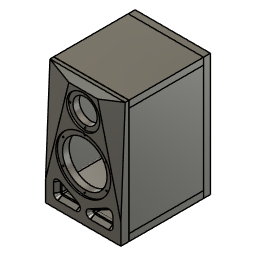
Spookers V2 v19 (Autodesk Fusion 360 design; units mm, degrees)
Autodesk Fusion 360 part; units mm, degrees
ref_plane "Arbeitsebene4" through (0, 0, 10) normal (0, 0, 1) x (1, 0, 0) in component "Front"
sketch "Skizze1" plane through (0, 0, 10) normal (0, 0, 1) x (1, 0, 0) in component "Front"
  line L0 (0, 0) -> (208, 0)
  line L1 (208, 0) -> (208, 338)
  line L2 (208, 338) -> (0, 338)
  line L3 (0, 338) -> (0, 0)
  line L4 (19, 319) -> (189, 319) construction
  line L5 (189, 319) -> (189, 19) construction
  line L6 (189, 19) -> (19, 19) construction
  line L7 (19, 19) -> (19, 319) construction
  line L8 (104, 0) -> (104, 338) construction
  circle A0 centre (104, 269.25) radius 33.5
  circle A1 centre (104, 269.25) radius 45.75
  circle A2 centre (104, 142.75) radius 75.75
  circle A3 centre (104, 142.75) radius 61.5
  line L9 (86.352941, 38.411765) -> (36.352941, 65.078431)
  line L10 (29, 60.666667) -> (29, 34)
  line L11 (34, 29) -> (84, 29)
  arc A4 (84, 29) -> (86.352941, 38.411765) centre (84, 34) ccw
  arc A5 (36.352941, 65.078431) -> (29, 60.666667) centre (34, 60.666667) ccw
  arc A6 (29, 34) -> (34, 29) centre (34, 34) ccw
  line L12 (121.647059, 38.411765) -> (171.647059, 65.078431)
  arc A7 (179, 60.666667) -> (171.647059, 65.078431) centre (174, 60.666667) ccw
  line L13 (179, 60.666667) -> (179, 34)
  arc A8 (174, 29) -> (179, 34) centre (174, 34) ccw
  line L14 (174, 29) -> (124, 29)
  arc A9 (121.647059, 38.411765) -> (124, 29) centre (124, 34) ccw
  circle A10 centre (104, 142.75) radius 69 construction
  circle A11 centre (104, 269.25) radius 41 construction
  circle A12 centre (104, 211.75) radius 2
  circle A13 centre (44.244247, 177.25) radius 2
  circle A14 centre (44.244247, 108.25) radius 2
  circle A15 centre (104, 73.75) radius 2
  circle A16 centre (163.755753, 108.25) radius 2
  circle A17 centre (163.755753, 177.25) radius 2
  circle A18 centre (104, 310.25) radius 2
  circle A19 centre (63, 269.25) radius 2
  circle A20 centre (104, 228.25) radius 2
  circle A21 centre (145, 269.25) radius 2
  point P0 (29, 69)
  point P1 (29, 29)
  dimension "d20" = 338
  dimension "d21" = 208
  dimension "d22" = 19
  dimension "d23" = 19
  dimension "d24" = 19
  dimension "d25" = 19
  dimension "d26" = 67
  dimension "d27" = 91.5
  dimension "d28" = 151.5
  dimension "d29" = 123
  dimension "d30" = 126.5
  dimension "d31" = 49.75
  dimension "d32" = 5
  dimension "d33" = 40
  dimension "d34" = 55
  dimension "d35" = 10
  dimension "d36" = 10
  dimension "d37" = 5
  dimension "d75" = 138
  dimension "d76" = 82
  dimension "d82" = 4
  dimension "d84" = 360
  dimension "d85" = 4
  dimension "d87" = 360
  constraint horizontal L0
  constraint vertical L1
  constraint horizontal L2
  constraint vertical L3
  constraint coincident L0.start L3.end
  constraint horizontal L4
  constraint vertical L5
  constraint horizontal L6
  constraint vertical L7
  constraint midpoint L0 L8.start
  constraint midpoint L2 L8.end
  constraint coincident L8 A0.centre
  constraint concentric A0 A1
  constraint coincident L8 A2.centre
  constraint concentric A2 A3
  constraint vertical L10
  constraint perpendicular L10 L11
  constraint tangent L11 A4
  constraint tangent L9 A4
  constraint coincident P0 L10
  constraint coincident P0 L9
  constraint tangent L10 A5
  constraint tangent L9 A5
  constraint coincident P1 L10
  constraint coincident P1 L11
  constraint tangent L10 A6
  constraint tangent L11 A6
  constraint equal A5 A6
  constraint symmetric L8 L11.end L14.end
  constraint symmetric L8 A4 A9
  constraint symmetric L8 A5 A7
  constraint symmetric L8 L10.end L13.end
  constraint symmetric L8 L11.start A8.start
  constraint symmetric L8 A6 A8
  constraint concentric A3 A10
  constraint concentric A1 A11
  constraint coincident A10 A12.centre
  constraint coincident L8 A12.centre
  constraint coincident A11 A18.centre
  constraint coincident L8 A18.centre
  measures "d20" distance of L0.start L2.end
  measures "d21" distance of L0.start L0.end
  measures "d22" distance of L0 L6
  measures "d23" distance of L3 L7
  measures "d24" distance of L2 L4
  measures "d25" distance of L1 L5
  measures "d26" diameter of A0
  measures "d27" diameter of A1
  measures "d28" diameter of A2
  measures "d29" diameter of A3
  measures "d30" distance of A0.centre A2.centre
  measures "d31" distance of L4 A0.centre
  measures "d32" radius of A4
  measures "d33" distance of P0 P1
  measures "d34" distance of P1 L11.end
  measures "d35" distance of L6 L11
  measures "d36" distance of L7 L10
  measures "d37" radius of A5
  measures "d75" diameter of A10
  measures "d76" diameter of A11
  measures "d82" diameter of A12
  measures "d85" diameter of A18
extrude "Extrusion1" add sketch "Skizze1" along normal blind 12 contours L0 L1 L2 L3 picked at (33.391134, 261.950937) makes body 1 in component "Front"
extrude "Extrusion2" add sketch "Skizze1" along normal up to surface (6.9 mm away) contours A1 picked at (110.51531, 230.025491) bodies 1 in component "Front"
extrude "Extrusion3" add sketch "Skizze1" along normal up to surface (7.7 mm away) contours A2 picked at (50.877626, 99.554747) bodies 1 in component "Front"
chamfer "Fase1" distance 7 distance2 12 12 edges at (59, 29, 22) (30.464466, 30.464466, 22) (29, 47.333333, 22) (31.427521, 64.954131, 22) (61.352941, 51.745098, 22) (88.850713, 32.787322, 22) (149, 29, 22) (119.149287, 32.787322, 22) (146.647059, 51.745098, 22) (176.572479, 64.954131, 22) (179, 47.333333, 22) (177.535534, 30.464466, 22) measured on face at (33.391134, 261.950937, 22) measured on face at (33.391134, 261.950937, 22) measured on face at (33.391134, 261.950937, 22) measured on face at (33.391134, 261.950937, 22) measured on face at (33.391134, 261.950937, 22) measured on face at (33.391134, 261.950937, 22) measured on face at (33.391134, 261.950937, 22) measured on face at (33.391134, 261.950937, 22) measured on face at (33.391134, 261.950937, 22) measured on face at (33.391134, 261.950937, 22) measured on face at (33.391134, 261.950937, 22) measured on face at (33.391134, 261.950937, 22) on bodies 1 in component "Front"
sketch "Skizze2" plane through (0, 0, 22) normal (0, 0, 1) x (1, 0, 0) in component "Front"
  circle A0 centre (104, 142.75) radius 75.75
  circle A1 centre (104, 269.25) radius 45.75
  line L0 (0, 338) -> (0, 0)
  line L1 (0, 0) -> (208, 0)
  line L2 (208, 0) -> (208, 338)
  line L3 (208, 338) -> (0, 338)
  line L4 (0, 320) -> (208, 320)
  line L5 (143.851304, 320) -> (208, 57.222965)
  line L6 (104, 338) -> (104, 0) construction
  line L7 (208, 338) -> (0, 338)
  line L8 (64.148696, 320) -> (0, 57.222965)
  line L9 (84, 22) -> (34, 22)
  arc A2 (22, 34) -> (34, 22) centre (34, 34) ccw
  line L10 (22, 34) -> (22, 60.666667)
  arc A3 (39.647059, 71.254902) -> (22, 60.666667) centre (34, 60.666667) ccw
  line L11 (39.647059, 71.254902) -> (89.647059, 44.588235)
  arc A4 (84, 22) -> (89.647059, 44.588235) centre (84, 34) ccw
  line L12 (174, 22) -> (124, 22)
  arc A5 (118.352941, 44.588235) -> (124, 22) centre (124, 34) ccw
  line L13 (118.352941, 44.588235) -> (168.352941, 71.254902)
  arc A6 (186, 60.666667) -> (168.352941, 71.254902) centre (174, 60.666667) ccw
  line L14 (186, 60.666667) -> (186, 34)
  arc A7 (174, 22) -> (186, 34) centre (174, 34) ccw
  point P0 (104, 269.25)
  point P1 (104, 142.75)
  dimension "d44" = 50.75
  dimension "d45" = 80.75
  dimension "d46" = 50.75
  constraint coincident L0 L4.start
  constraint coincident L2 L4.end
  constraint perpendicular L2 L4
  constraint midpoint L3 L6.start
  constraint coincident L1 L6.end
  constraint perpendicular L6 L7
  measures "d44" distance of L5 P0
  measures "d45" distance of L5 P1
  measures "d46" distance of L4 P0
ref_plane "Arbeitsebene1" through (143.851304, 320, 22) normal (0.17229751, 0.04206098, 0.98414655) x (-0.23715415, 0.97147203, 0) in component "Front"
ref_plane "Arbeitsebene2" through (0, 320, 22) normal (0, 0.5547002, 0.83205029) x (-1, 0, 0) in component "Front"
ref_plane "Arbeitsebene3" through (64.148696, 320, 22) normal (0.17229751, -0.04206098, -0.98414655) x (0.23715415, 0.97147203, 0) in component "Front"
split "Teilen1" by plane through (143.851304, 320, 22) normal (0.17229751, 0.04206098, 0.98414655) bodies 1 makes body 2 at (185.152391, 244.407655, 22) in component "Front"
split "Teilen2" by plane through (64.148696, 320, 22) normal (0.17229751, -0.04206098, -0.98414655) bodies 1 makes body 3 at (14.081416, 171.75, 10) in component "Front"
split "Teilen3" by plane through (0, 320, 22) normal (0, 0.5547002, 0.83205029) bodies 3 makes body 4 at (92.180942, 338, 14) in component "Front"
delete_body "Körper entfernen1" bodies 1 in component "Front"
delete_body "Körper entfernen2" bodies 2 in component "Front"
delete_body "Körper entfernen3" bodies 4 in component "Front"
extrude "Extrusion4" add sketch "Skizze1" against normal blind 10.5 contours L0 L1 L2 L3 | A1 | A2 picked at (33.391134, 261.950937) picked at (110.51531, 230.025491) picked at (50.877626, 99.554747) bodies 3 in component "Front"
sketch "Skizze1 (2)" plane through (0, 0, 0) normal (0, 0, 1) x (1, 0, 0) in component "Seiten"
  line L0 (0, 0) -> (208, 0) construction
  line L1 (208, 0) -> (208, 19) construction
  line L2 (208, 19) -> (0, 19) construction
  line L3 (0, 19) -> (0, 0) construction
  line L4 (0, 19) -> (19, 19)
  line L5 (19, 19) -> (19, 319)
  line L6 (19, 319) -> (0, 319)
  line L7 (0, 319) -> (0, 19)
  line L8 (208, 19) -> (189, 19)
  line L9 (189, 19) -> (189, 319)
  line L10 (189, 319) -> (208, 319)
  line L11 (208, 319) -> (208, 19)
  dimension "d52" = 208
  dimension "d53" = 19
  dimension "d54" = 19
  dimension "d55" = 300
  dimension "d56" = 19
  dimension "d57" = 300
  constraint horizontal L0
  constraint vertical L1
  constraint horizontal L2
  constraint vertical L3
  constraint coincident L0.start L3.end
  constraint horizontal L4
  constraint vertical L5
  constraint horizontal L6
  constraint vertical L7
  constraint horizontal L8
  constraint vertical L9
  constraint horizontal L10
  constraint vertical L11
  measures "d52" distance of L0.start L0.end
  measures "d53" distance of L0.start L2.end
  measures "d54" distance of L2.end L4.end
  measures "d55" distance of L2.end L6.end
  measures "d56" distance of L1.end L8.end
  measures "d57" distance of L1.end L10.end
extrude "Extrusion1'" add sketch "Skizze1 (2)" against normal blind 206.27451 separate body contours L4 L5 L6 L7 | L8 L9 L10 L11 picked at (6.333333, 219) picked at (195.333333, 119) makes body 5 at (189, 119, -68.75817) makes body 6 at (0, 219, -68.75817) in component "Seiten"
sketch "Skizze1 (3)" plane through (0, 0, 0) normal (0, 0, 1) x (1, 0, 0) in component "Oben/Unten"
  line L0 (0, 0) -> (208, 0)
  line L1 (208, 0) -> (208, 19)
  line L2 (208, 19) -> (0, 19)
  line L3 (0, 19) -> (0, 0)
  line L4 (0, 19) -> (0, 319) construction
  line L5 (0, 319) -> (208, 319)
  line L6 (208, 319) -> (208, 338)
  line L7 (208, 338) -> (0, 338)
  line L8 (0, 338) -> (0, 319)
  dimension "d60" = 208
  dimension "d61" = 19
  dimension "d62" = 300
  dimension "d63" = 208
  dimension "d64" = 19
  constraint horizontal L0
  constraint vertical L1
  constraint horizontal L2
  constraint vertical L3
  constraint coincident L0.start L3.end
  constraint perpendicular L2 L4
  constraint horizontal L5
  constraint vertical L6
  constraint horizontal L7
  constraint vertical L8
  measures "d60" distance of L0.start L0.end
  measures "d61" distance of L0.start L2.end
  measures "d62" distance of L2.end L4.end
  measures "d63" distance of L4.end L5.end
  measures "d64" distance of L4.end L7.end
extrude "Extrusion1''" add sketch "Skizze1 (3)" against normal blind 206.27451 separate body contours L0 L1 L2 L3 | L5 L6 L7 L8 picked at (69.333333, 12.666667) picked at (69.333333, 325.333333) makes body 7 at (138.666667, 19, -137.51634) makes body 8 at (138.666667, 338, -137.51634) in component "Oben/Unten"
ref_plane "Arbeitsebene1" through (0, 0, -206.27451) normal (0, 0, 1) x (1, 0, 0) in component "Hinten"
sketch "Skizze1 (4)" plane through (0, 0, -206.27451) normal (0, 0, 1) x (1, 0, 0) in component "Hinten"
  line L0 (0, 0) -> (208, 0)
  line L1 (208, 0) -> (208, 338)
  line L2 (208, 338) -> (0, 338)
  line L3 (0, 338) -> (0, 0)
  dimension "d68" = 208
  dimension "d69" = 338
  constraint horizontal L0
  constraint vertical L1
  constraint horizontal L2
  constraint vertical L3
  constraint coincident L0.start L3.end
  measures "d68" distance of L0.start L0.end
  measures "d69" distance of L0.start L2.end
extrude "Extrusion1'''" add sketch "Skizze1 (4)" against normal blind 19 separate body contours L0 L1 L2 L3 picked at (69.333333, 112.666667) makes body 9 in component "Hinten"
ref_plane "Arbeitsebene5" through (121.647059, 38.411765, 10) normal (0, 0, 1) x (1, 0, 0) in component "Front"
sketch "Skizze4" plane through (121.647059, 38.411765, 10) normal (0, 0, 1) x (1, 0, 0) in component "Front"
  arc A0 (57.352941, 22.254902) -> (50, 26.666667) centre (52.352941, 22.254902) ccw
  line L0 (50, 26.666667) -> (0, 0)
  arc A1 (0, 0) -> (2.352941, -9.411765) centre (2.352941, -4.411765) ccw
  line L1 (2.352941, -9.411765) -> (52.352941, -9.411765)
  arc A2 (52.352941, -9.411765) -> (57.352941, -4.411765) centre (52.352941, -4.411765) ccw
  line L2 (57.352941, -4.411765) -> (57.352941, 22.254902)
  circle A3 centre (-77.402812, 69.838235) radius 2
  circle A4 centre (-77.402812, 138.838235) radius 2
  circle A5 centre (42.108694, 69.838235) radius 2
  circle A6 centre (-17.647059, 189.838235) radius 2
  circle A7 centre (23.352941, 230.838235) radius 2
  circle A8 centre (-17.647059, 230.838235) radius 33.5
  circle A9 centre (-17.647059, 271.838235) radius 2
  arc A10 (-92.647059, -4.411765) -> (-87.647059, -9.411765) centre (-87.647059, -4.411765) ccw
  line L3 (-87.647059, -9.411765) -> (-37.647059, -9.411765)
  arc A11 (-37.647059, -9.411765) -> (-35.294118, 0) centre (-37.647059, -4.411765) ccw
  line L4 (-35.294118, 0) -> (-85.294118, 26.666667)
  arc A12 (-85.294118, 26.666667) -> (-92.647059, 22.254902) centre (-87.647059, 22.254902) ccw
  line L5 (-92.647059, 22.254902) -> (-92.647059, -4.411765)
  circle A13 centre (42.108694, 138.838235) radius 2
  circle A14 centre (-58.647059, 230.838235) radius 2
  circle A15 centre (-17.647059, 173.338235) radius 2
  circle A16 centre (-17.647059, 104.338235) radius 61.5
  circle A17 centre (-17.647059, 35.338235) radius 2
  line L6 (-121.647059, -38.411765) -> (-121.647059, 299.588235)
  line L7 (-121.647059, 299.588235) -> (86.352941, 299.588235)
  line L8 (86.352941, 299.588235) -> (86.352941, -38.411765)
  line L9 (86.352941, -38.411765) -> (-121.647059, -38.411765)
  line L10 (2.352941, -7.411765) -> (52.352941, -7.411765)
  arc A18 (52.352941, -7.411765) -> (55.352941, -4.411765) centre (52.352941, -4.411765) ccw
  line L11 (55.352941, -4.411765) -> (55.352941, 22.254902)
  arc A19 (55.352941, 22.254902) -> (50.941176, 24.901961) centre (52.352941, 22.254902) ccw
  line L12 (50.941176, 24.901961) -> (0.941176, -1.764706)
  arc A20 (0.941176, -1.764706) -> (2.352941, -7.411765) centre (2.352941, -4.411765) ccw
  line L13 (-90.647059, 22.254902) -> (-90.647059, -4.411765)
  arc A21 (-90.647059, -4.411765) -> (-87.647059, -7.411765) centre (-87.647059, -4.411765) ccw
  line L14 (-87.647059, -7.411765) -> (-37.647059, -7.411765)
  arc A22 (-37.647059, -7.411765) -> (-36.235294, -1.764706) centre (-37.647059, -4.411765) ccw
  line L15 (-36.235294, -1.764706) -> (-86.235294, 24.901961)
  arc A23 (-86.235294, 24.901961) -> (-90.647059, 22.254902) centre (-87.647059, 22.254902) ccw
  dimension "d107" = -2
  dimension "d119" = -2
extrude "Extrusion5" add sketch "Skizze4" against normal blind 126.1 separate body contours A0 L0 A1 L1 A2 L2 | A10 L3 A11 L4 A12 L5 picked at (33.647059, 17.189542) picked at (-69.254902, 16.601307) makes body 10 at (154.980392, 56.189542, -32.033333) makes body 11 at (69.686275, 47.300654, -74.066667) in component "Front"
chamfer "Fase2" distance 2 angle 45 6 edges at (147.588235, 49.980392, 10) (175.543487, 63.239145, 10) (177, 47.333333, 10) (176.12132, 31.87868, 10) (149, 31, 10) (121.089572, 33.272393, 10) on bodies 10 11 in component "Front"
chamfer "Fase2" distance 2 angle 45 6 edges at (59, 31, 10) (31.87868, 31.87868, 10) (31, 47.333333, 10) (32.456513, 63.239145, 10) (60.411765, 49.980392, 10) (86.910428, 33.272393, 10) on bodies 10 11 in component "Front"
sketch "Skizze5" plane through (0, 0, -116.1) normal (0, 0, -1) x (-1, 0, 0) in component "Front"
  arc A0 (-124, 31) -> (-122.588235, 36.647059) centre (-124, 34) ccw
  line L0 (-124, 31) -> (-174, 31)
  line L1 (-177, 34) -> (-177, 60.666667)
  arc A1 (-172.588235, 63.313725) -> (-177, 60.666667) centre (-174, 60.666667) ccw
  line L2 (-172.588235, 63.313725) -> (-122.588235, 36.647059)
  line L3 (-179, 60.666667) -> (-179, 34)
  arc A2 (-179, 34) -> (-174, 29) centre (-174, 34) ccw
  line L4 (-174, 29) -> (-124, 29)
  arc A3 (-124, 29) -> (-121.647059, 38.411765) centre (-124, 34) ccw
  line L5 (-121.647059, 38.411765) -> (-171.647059, 65.078431)
  arc A4 (-171.647059, 65.078431) -> (-179, 60.666667) centre (-174, 60.666667) ccw
  arc A5 (-177, 34) -> (-174, 31) centre (-174, 34) ccw
  line L6 (-186, 60.666667) -> (-186, 34)
  arc A6 (-186, 34) -> (-174, 22) centre (-174, 34) ccw
  line L7 (-174, 22) -> (-124, 22)
  arc A7 (-124, 22) -> (-118.352941, 44.588235) centre (-124, 34) ccw
  line L8 (-118.352941, 44.588235) -> (-168.352941, 71.254902)
  arc A8 (-168.352941, 71.254902) -> (-186, 60.666667) centre (-174, 60.666667) ccw
  dimension "d113" = 7
sketch "Skizze6" plane through (0, 0, -116.1) normal (0, 0, -1) x (-1, 0, 0) in component "Front"
  arc A0 (-31, 60.666667) -> (-35.411765, 63.313725) centre (-34, 60.666667) ccw
  line L0 (-31, 60.666667) -> (-31, 34)
  arc A1 (-34, 31) -> (-31, 34) centre (-34, 34) ccw
  line L1 (-34, 31) -> (-84, 31)
  arc A2 (-85.411765, 36.647059) -> (-84, 31) centre (-84, 34) ccw
  line L2 (-85.411765, 36.647059) -> (-35.411765, 63.313725)
  line L3 (-29, 34) -> (-29, 60.666667)
  arc A3 (-29, 60.666667) -> (-36.352941, 65.078431) centre (-34, 60.666667) ccw
  line L4 (-36.352941, 65.078431) -> (-86.352941, 38.411765)
  arc A4 (-86.352941, 38.411765) -> (-84, 29) centre (-84, 34) ccw
  line L5 (-84, 29) -> (-34, 29)
  arc A5 (-34, 29) -> (-29, 34) centre (-34, 34) ccw
extrude "Extrusion6" add sketch "Skizze5" against normal blind 10 contours L6 A6 L7 A7 L8 A8 picked at (-137.215686, 49.359477) bodies 10 in component "Front"
extrude "Extrusion7" add sketch "Skizze6" against normal blind 2 contours A0 L0 A1 L1 A2 L2 picked at (-51.607843, 43.653595) bodies 11 in component "Front"
fillet "Abrundung1" radius 4 24 edges at (149, 31, -116.1) (176.12132, 31.87868, -116.1) (177, 47.333333, -116.1) (175.543487, 63.239145, -116.1) (147.588235, 49.980392, -116.1) (121.089572, 33.272393, -116.1) (186, 47.333333, -116.1) (182.485281, 25.514719, -116.1) (149, 22, -116.1) (112.35829, 31.089572, -116.1) (143.352941, 57.921569, -116.1) (180.173949, 70.956582, -116.1) (149, 22, -106.1) (182.485281, 25.514719, -106.1) (186, 47.333333, -106.1) (180.173949, 70.956582, -106.1) (143.352941, 57.921569, -106.1) (112.35829, 31.089572, -106.1) (149, 29, -106.1) (177.535534, 30.464466, -106.1) (179, 47.333333, -106.1) (176.572479, 64.954131, -106.1) (146.647059, 51.745098, -106.1) (119.149287, 32.787322, -106.1) on bodies 10 in component "Front"
move_body "Verschieben1" [rolled back] in component "Front"
move_body "Verschieben2" [rolled back] rotate angle -90 in component "Front"
component "Front" placed x (1, 0, 0) y (0, 1, 0) z (0, 0, 1) at (0, 0, 0)
component "Seiten" placed x (1, 0, 0) y (0, 1, 0) z (0, 0, 1) at (0, 0, 0)
component "Oben/Unten" placed x (1, 0, 0) y (0, 1, 0) z (0, 0, 1) at (0, 0, 0)
component "Hinten" placed x (1, 0, 0) y (0, 1, 0) z (0, 0, 1) at (0, 0, 0)
equation "VolumenBox = 10 l"
equation "VolumenLautsprecher = 0.32 l"
equation "VolumenPorts = 0.2 l"
equation "VolumenGesamt = VolumenBox + VolumenLautsprecher + VolumenPorts"
equation "MaterialDicke = 19 mm"
equation "Höhe = 300 mm"
equation "Breite = 170 mm"
equation "Tiefe = VolumenGesamt / ( Höhe * Breite )"
equation "HochtönerEinbauloch = 67 mm"
equation "HochtönerFlushmountDurchmesser = 91.5 mm"
equation "HochtönerEinbauTiefe = 5.1 mm"
equation "TieftönerEinbauloch = 123 mm"
equation "TieftönerFlushmountDurchmesser = 151.5 mm"
equation "TieftönerEinbauTiefe = 4.3 mm"
equation "Knickabstand = 5 mm"
equation "PortBreite = 55 mm"
equation "Porthöhe1 = 40 mm"
equation "Porthöhe2 = 10 mm"
equation "Portabstand = 10 mm"
equation "d20 = Höhe + 2 * MaterialDicke"
equation "d21 = Breite + 2 * MaterialDicke"
equation "d22 = MaterialDicke"
equation "d23 = MaterialDicke"
equation "d24 = MaterialDicke"
equation "d25 = MaterialDicke"
equation "d26 = HochtönerEinbauloch"
equation "d27 = HochtönerFlushmountDurchmesser"
equation "d28 = TieftönerFlushmountDurchmesser"
equation "d29 = TieftönerEinbauloch"
equation "d30 = HochtönerFlushmountDurchmesser / 2 + TieftönerFlushmountDurchmesser / 2 + 5 mm"
equation "d31 = HochtönerFlushmountDurchmesser / 2 + 4 mm"
equation "d32 = Porthöhe2 / 2"
equation "d33 = Porthöhe1"
equation "d34 = PortBreite"
equation "d35 = Portabstand"
equation "d36 = Portabstand"
equation "d37 = Porthöhe2 / 2"
equation "d38 = ( MatterialFront - ( MatterialFront - TiefeAnschrägung ) )"
equation "d40 = -HochtönerEinbauTiefe"
equation "d42 = -TieftönerEinbauTiefe"
equation "d44 = HochtönerFlushmountDurchmesser / 2 + Knickabstand"
equation "d45 = TieftönerFlushmountDurchmesser / 2 + Knickabstand"
equation "d46 = HochtönerFlushmountDurchmesser / 2 + Knickabstand"
equation "d52 = Breite + 2 * MaterialDicke"
equation "d53 = MaterialDicke"
equation "d54 = MaterialDicke"
equation "d55 = Höhe"
equation "d56 = MaterialDicke"
equation "d57 = Höhe"
equation "d58 = -Tiefe"
equation "d60 = Breite + 2 * MaterialDicke"
equation "d61 = MaterialDicke"
equation "d62 = Höhe"
equation "d63 = Breite + 2 * MaterialDicke"
equation "d64 = MaterialDicke"
equation "d65 = -Tiefe"
equation "d67 = -Tiefe"
equation "d68 = Breite + 2 * MaterialDicke"
equation "d69 = Höhe + 2 * MaterialDicke"
equation "d70 = -MaterialDicke"
equation "d73 = -( MatterialFront - TiefeAnschrägung )"
equation "d75 = TieftönerBoltcircle"
equation "d76 = HochtönerBoltcircle"
equation "SchraubLöcher = 4 mm"
equation "TieftönerBoltcircle = 138 mm"
equation "HochtönerBoltcircle = 82 mm"
equation "TieftönerLochanzahl = 6"
equation "HochtönerLochanzahl = 4"
equation "d82 = SchraubLöcher"
equation "d83 = TieftönerLochanzahl"
equation "d85 = SchraubLöcher"
equation "d86 = HochtönerLochanzahl"
equation "MatterialFront = 22.5 mm"
equation "TiefeAnschrägung = 12 mm"
equation "Portlänge = 126.1 mm"
equation "d108 = -Portlänge"
